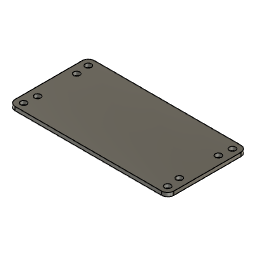
Platform_ top (Autodesk Fusion 360 design; units mm, degrees)
Autodesk Fusion 360 part; units mm, degrees
sketch "Sketch1" plane through (0, 0, 0) normal (0, 0, 1) x (1, 0, 0)
  line L0 (-65, -27.5) -> (-65, 27.5)
  arc A0 (-60, 32.5) -> (-65, 27.5) centre (-60, 27.5) ccw
  arc A1 (-65, -27.5) -> (-60, -32.5) centre (-60, -27.5) ccw
  circle A2 centre (-59, 26.5) radius 2.5
  circle A3 centre (-59, -26.5) radius 2.5
  line L1 (0, 32.5) -> (0, -32.5) construction
  line L2 (-60, 32.5) -> (0, 32.5)
  line L3 (-60, -32.5) -> (0, -32.5)
  circle A4 centre (-58, 16) radius 2.5
  circle A5 centre (-58, -16) radius 2.5
  circle A6 centre (58, -16) radius 2.5
  arc A7 (60, -32.5) -> (65, -27.5) centre (60, -27.5) ccw
  line L4 (60, 32.5) -> (0, 32.5)
  circle A8 centre (59, 26.5) radius 2.5
  circle A9 centre (59, -26.5) radius 2.5
  line L5 (65, -27.5) -> (65, 27.5)
  arc A10 (65, 27.5) -> (60, 32.5) centre (60, 27.5) ccw
  circle A11 centre (58, 16) radius 2.5
  line L6 (60, -32.5) -> (0, -32.5)
  dimension "d1" = 65
  dimension "d5" = 5
  dimension "d6" = 5
  dimension "d9" = 5
  dimension "d11" = 6
  dimension "d12" = 5
  dimension "d14" = 6
  dimension "d21" = 7
  dimension "d22" = 7
  dimension "d23" = 32
  dimension "d24" = 16.5
  dimension "d25" = 65
  dimension "d28" = 5
  dimension "d29" = 5
  constraint vertical L0
  constraint tangent L0 A0
  constraint tangent L0 A1
  constraint tangent A0 L2
  constraint tangent A1 L3
  constraint symmetric A0.start L1 L4.start
  constraint symmetric L0.end L1 L5.end
  constraint symmetric A0 L1 A10
  constraint symmetric A1.end L1 A7.start
  constraint symmetric L0.start L1 A7.end
  constraint symmetric A1 L1 A7
  constraint symmetric A2 L1 A8
  constraint symmetric A3 L1 A9
  constraint symmetric L2.end L1 L4.end
  constraint symmetric L3.end L1 L6.end
  constraint symmetric L1 A4 A11
  constraint symmetric L1 A5 A6
  measures "d1" distance of origin L0
  measures "d5" radius of A0
  measures "d6" radius of A1
  measures "d9" diameter of A2
  measures "d11" distance of L0 A2.centre
  measures "d12" diameter of A3
  measures "d14" distance of L0 A3.centre
  measures "d21" distance of L0 A4.centre
  measures "d22" distance of L0 A5.centre
  measures "d23" distance of A4.centre A5.centre
  measures "d24" distance of L2 A4.centre
  measures "d25" distance of L2 L3
  measures "d28" diameter of A4
  measures "d29" diameter of A5
extrude "Extrude1" add sketch "Sketch1" along normal blind 3
equation "d6 = d5"
equation "d12 = d9"
equation "d14 = d11"
equation "d22 = d21"
equation "d24 = ( d25 - d23 ) / 2"
equation "d29 = d28"
